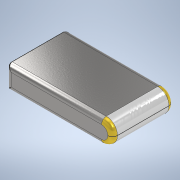
# Autodesk Inventor part: LiPo Battery
Saved by Autodesk Inventor 2022 (Build 260153000, 153)
## iProperties
Created: 2021-10-21
Part Number: LiPo Battery
Material: Generic
Document SubType Name: Modeling
Designer: dech3
Density: 1 g/cm^3
Appearance: Default
Author: dech3
Autodesk Inventor part; units mm, degrees
ref_plane "YZ Plane" through (0, 0, 0) normal (1, 0, 0) x (0, 1, 0)
ref_plane "XZ Plane" through (0, 0, 0) normal (0, 1, 0) x (-1, 0, 0)
ref_plane "XY Plane" through (0, 0, 0) normal (0, 0, 1) x (1, 0, 0)
sketch "Sketch1" plane through (0, 0, 0) normal (0, 1, 0) x (-1, 0, 0)
  line L0 (22, -12.65) -> (-22, -12.65)
  line L1 (-22, -12.65) -> (-22, 12.65)
  line L2 (-22, 12.65) -> (22, 12.65)
  line L3 (22, 12.65) -> (22, -12.65)
  point P0 (0, 0)
  dimension "d0" = 44
  dimension "d2" = 22
  dimension "d3" = 25.3
  dimension "d4" = 12.65
  constraints: 8 end point, 2 parallel, 1 horizontal, 1 perpendicular
  measures "d0" distance between parallel lines of L1 L3
  measures "d2" distance from line of L3 point (0, 0)
  measures "d3" distance between parallel lines of L2 L0
  measures "d4" distance from line of point (0, 0) L0
extrude "Extrusion1" add sketch "Sketch1" along normal blind 9.32
fillet "Fillet1" radius 4.6 2 edges at (22, 9.32, 0) (22, 0, 0)
fillet "Fillet2" radius 0.5 2 edges at (-22, 9.32, 0) (-22, 0, 0)
fillet "Fillet3" radius 2 16 edges at (20.6527, 7.9727, 12.65) (22, 4.66, 12.65) (20.6527, 1.3473, 12.65) (-2.05, 0, 12.65) (-21.8536, 0.1464, 12.65) (-22, 4.66, 12.65) (-21.8536, 9.1736, 12.65) (-2.05, 9.32, 12.65) (-21.8536, 9.1736, -12.65) (-22, 4.66, -12.65) (-21.8536, 0.1464, -12.65) (-2.05, 0, -12.65) (20.6527, 1.3473, -12.65) (22, 4.66, -12.65) (20.6527, 7.9727, -12.65) (-2.05, 9.32, -12.65)
equation "\"d2\" = 0.5 * d0"
equation "\"d4\" = 0.5 * d3"
body "Solid1"
